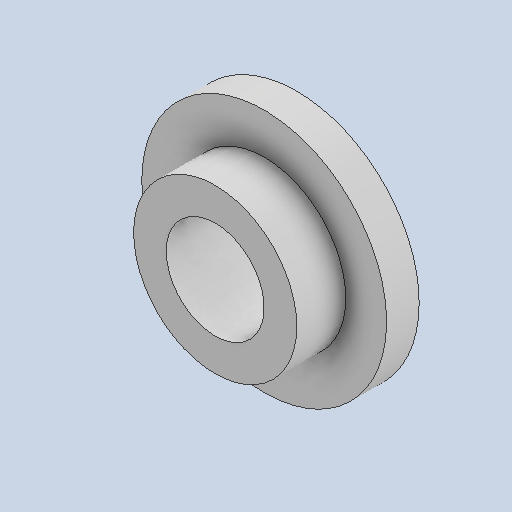
# Autodesk Inventor part: 10mm_bearing
Saved by Autodesk Inventor 2024.3 (Build 283343000, 343)
## iProperties
Created: 2024-12-09
Part Number: 10mm_bearing
Material: 一般
Document SubType Name: Modeling
Designer: 佐藤智貴
Density: 1 g/cm^3
Appearance: 既定
Mass: 1.61588 g
Surface Area: 7.3042 cm^2
Volume: 0.598473 cm^3
Author: 佐藤智貴
Autodesk Inventor part; units mm, degrees
ref_plane "YZ Plane" through (0, 0, 0) normal (1, 0, 0) x (0, 1, 0)
ref_plane "XZ Plane" through (0, 0, 0) normal (0, 1, 0) x (-1, 0, 0)
ref_plane "XY Plane" through (0, 0, 0) normal (0, 0, 1) x (1, 0, 0)
sketch "スケッチ1" plane through (0, 0, 0) normal (0, 0, 1) x (1, 0, 0)
  circle A0 centre (0, 0) radius 5
  circle A1 centre (0, 0) radius 7.5
  dimension "d0" = 10
  dimension "d1" = 15
  constraints: 2 centre point, 1 coincident
  measures "d0" diameter of A0
  measures "d1" diameter of A1
extrude "押し出し1" add sketch "スケッチ1" along normal blind 8 contours A0 | A1
sketch "スケッチ2" plane through (0, 0, 8) normal (0, 0, 1) x (1, 0, 0)
  circle A0 centre (0, 0) radius 5
  circle A1 centre (0, 0) radius 3
  circle A2 centre (0, 0) radius 10
  dimension "d4" = 10
  dimension "d5" = 6
  dimension "d8" = 20
  constraints: 3 centre point, 2 coincident
  measures "d4" diameter of A0
  measures "d5" diameter of A1
  measures "d8" diameter of A2
extrude "押し出し2" cut sketch "スケッチ2" against normal blind 6
sketch "スケッチ4" plane through (0, 0, 2) normal (0, 0, 1) x (1, 0, 0)
  circle A0 centre (0, 0) radius 3
  constraints: 1 centre point, 1 coincident
extrude "押し出し4" cut sketch "スケッチ4" against normal blind 5
sketch "スケッチ5" plane through (0, 0, 8) normal (0, 0, 1) x (1, 0, 0)
  circle A0 centre (0, 0) radius 10.699
  constraints: 1 centre point, 1 coincident
extrude "押し出し5" cut sketch "スケッチ5" against normal blind 3
